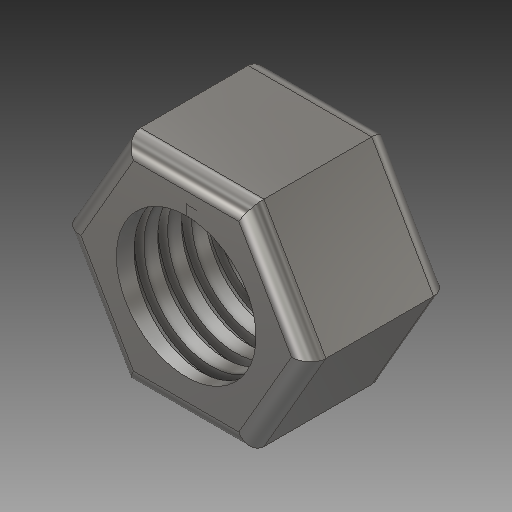
# Autodesk Inventor part: Tuerca
Saved by Autodesk Inventor 2019 (Build 230136000, 136)
## iProperties
Created: 2020-02-22
Part Number: Tuerca
Material: Stainless Steel
Document SubType Name: Modeling
Designer: Elías Sánchez
Density: 8 g/cm^3
Appearance: Semi-Polished
Description: Cemaco
Author: Elías Sánchez
Revision Number: IR
Autodesk Inventor part; units mm, degrees
ref_plane "YZ Plane" through (0, 0, 0) normal (1, 0, 0) x (0, 1, 0)
ref_plane "XZ Plane" through (0, 0, 0) normal (0, 1, 0) x (-1, 0, 0)
ref_plane "XY Plane" through (0, 0, 0) normal (0, 0, 1) x (1, 0, 0)
sketch "Sketch1" plane through (0, 0, 0) normal (0, 0, 1) x (1, 0, 0)
  line L0 (6.2, 0) -> (3.1, -5.3694)
  line L1 (3.1, -5.3694) -> (-3.1, -5.3694)
  line L2 (-3.1, -5.3694) -> (-6.2, 0)
  line L3 (-6.2, 0) -> (-3.1, 5.3694)
  line L4 (-3.1, 5.3694) -> (3.1, 5.3694)
  line L5 (3.1, 5.3694) -> (6.2, 0)
  point P0 (0, 0)
  point P1 (0, 0)
  dimension "d0" = 12.4
  dimension "d1" = 5.3694
  constraints: 12 end point, 1 coincident, 13 other
  measures "d0" distance of L2.end L0.start
  measures "d1" vertical distance of L4.end L0.start
extrude "Extrusion1" add sketch "Sketch1" along normal blind 7
sketch "Sketch2" plane through (0, 0, 7) normal (0, 0, 1) x (1, 0, 0)
  circle A0 centre (0, 0) radius 3.5
  dimension "d4" = 7
  constraints: 1 centre point, 1 coincident
  measures "d4" diameter of A0
extrude "Extrusion2" cut sketch "Sketch2" against normal blind 7
fillet "Fillet1" radius 0.8 12 edges at (4.65, 2.6847, 7) (0, 5.3694, 7) (-4.65, 2.6847, 7) (-4.65, -2.6847, 7) (0, -5.3694, 7) (4.65, -2.6847, 7) (4.65, 2.6847, 0) (0, 5.3694, 0) (4.65, -2.6847, 0) (0, -5.3694, 0) (-4.65, -2.6847, 0) (-4.65, 2.6847, 0)
sketch "Sketch3" plane through (0, 0, 0) normal (1, 0, 0) x (0, 1, 0)
  line L0 (3.5, 7) -> (3.5, 0) projected
  line L1 (3.5, 7) -> (4, 7)
  line L2 (4, 7) -> (4, 6.5)
  line L3 (4, 6.5) -> (3.5, 6.5)
  line L4 (3.5, 6.5) -> (3.5, 7)
  point P0 (0, 0)
  dimension "d8" = 0.5
  dimension "d9" = 0.5
  constraints: 8 end point, 2 parallel, 1 horizontal, 1 perpendicular
  measures "d8" distance of L2.end L3.end
  measures "d9" distance of L1.end L2.end
coil "Coil1" sketch "Sketch3" operation cut axis through (0, 0, -10) along (0, 0, -1) pitch 1.1885 turns 5.89 hand right
body "Solid1"
